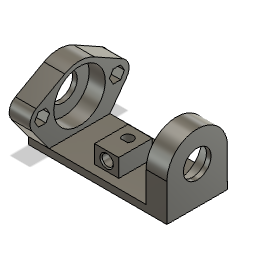
arm (Autodesk Fusion 360 design; units mm, degrees)
Autodesk Fusion 360 part; units mm, degrees
note: some values were not read from the file. Set by a fixed rule: which sketch regions a step uses.
sketch "Esquisse1" plane through (0, 0, 0) normal (0, 1, 0) x (1, 0, 0)
  circle A0 centre (0, 0) radius 2.25
  line L0 (30, -13.15) -> (-30, -13.15)
  line L1 (-30, -13.15) -> (-30, 13.15)
  line L2 (-30, 13.15) -> (30, 13.15)
  line L3 (30, 13.15) -> (30, -13.15)
  line L4 (30, -13.15) -> (-30, 13.15) construction
  line L5 (-30, -13.15) -> (30, 13.15) construction
  line L6 (-30, 13.15) -> (-21, 13.15)
  line L7 (-21, -13) -> (-30, -13)
  line L8 (-30, -13) -> (-30, 13.15)
  line L9 (0, 0) -> (0, -1.75) construction
  line L10 (0, -1.75) -> (1.4142, -1.75)
  line L11 (0, -1.75) -> (-1.4142, -1.75)
  dimension "d9" = 4.5
  dimension "d10" = 60
  dimension "d11" = 26.3
  dimension "d101" = 1.75
  constraint coincident A0.centre L9.start
  constraint horizontal L0
  constraint perpendicular L0 L1
  constraint parallel L0 L2
  constraint parallel L1 L3
  constraint coincident L4 A0.centre
  constraint coincident L5 A0.centre
  constraint horizontal L6
  constraint horizontal L7
  constraint vertical L8
  constraint vertical L9
  constraint coincident A0 L10.end
  constraint perpendicular L9 L10
  constraint symmetric L10.start L9 L11.start
  constraint symmetric L9 L10.end L11.end
  measures "d9" diameter of A0
  measures "d10" distance of L1.end L2.end
  measures "d11" distance of L0.end L1.end
  measures "d101" distance of A0.centre L9.end
ref_plane "Plan de construction1" through (30, 0, 0) normal (-1, 0, 0) x (0, 0, 1)
sketch "Esquisse2" plane through (30, 0, 0) normal (-1, 0, 0) x (0, 0, -1)
  line L0 (13, 0) -> (13, -20)
  line L1 (13.15, 0) -> (-13.15, 0)
  line L2 (-13.15, 0) -> (-13.15, -21)
  line L3 (0, 0) -> (0, -2) construction
  circle A0 centre (0, -13.15) radius 11.15
  circle A1 centre (0, -13.15) radius 6
  circle A2 centre (0, -13.15) radius 13.15
  dimension "d102" = 2
  dimension "d103" = 22.3
  dimension "d104" = 12
  dimension "d105" = 2
  constraint vertical L0
  constraint coincident L1.end L2.start
  constraint perpendicular L1 L2
  constraint coincident L3.start origin
  constraint perpendicular L1 L3
  constraint coincident L3.end A0
  constraint concentric A0 A1
  measures "d102" distance of L3.start L3.end
  measures "d103" diameter of A0
  measures "d104" diameter of A1
extrude "Extrusion1" add sketch "Esquisse2" along normal blind 9 contours L0 L1 A2 | L0 A2 | L1 L2 A2 picked at (12.3833, -13.15) makes body 1
extrude "Extrusion2" add sketch "Esquisse2" along normal blind 2 contours A0 bodies 1
ref_plane "Plan de construction2" through (-30, 0, 0) normal (1, 0, 0) x (0, 0, -1)
sketch "Esquisse16" plane through (-30, 0, 0) normal (1, 0, 0) x (0, 0, -1)
  circle A0 centre (0, 13.15) radius 13.15
  circle A1 centre (0, 13.15) radius 11.15
  circle A2 centre (0, 13.15) radius 6
  line L0 (13, 0) -> (13, 20)
  line L1 (-13.15, 0) -> (-13.15, 21)
  circle A3 centre (0, 13.15) radius 16.22 construction
  line L2 (0, 13.15) -> (-16.22, 13.15) construction
  line L3 (0, 13.15) -> (0, 29.37) construction
  circle A4 centre (-16.22, 13.15) radius 1.75
  circle A5 centre (-16.22, 13.15) radius 5.25
  circle A6 centre (16.22, 13.15) radius 5.25
  circle A7 centre (16.22, 13.15) radius 1.75
  line L4 (-13.15, 0) -> (-24.7417, 15.943)
  line L5 (0.9315, 28.726) -> (-24.187, 14.7182)
  line L6 (-0.9315, 28.726) -> (24.187, 14.7182)
  line L7 (13.15, 0) -> (24.7417, 15.943)
  line L8 (13.15, 0) -> (-13.15, 0)
  line L9 (-12.97, 13.1564) -> (-14.6006, 15.9678)
  line L10 (-14.6006, 15.9678) -> (-17.8506, 15.9614)
  line L11 (-17.8506, 15.9614) -> (-19.47, 13.1436)
  line L12 (-19.47, 13.1436) -> (-17.8394, 10.3322)
  line L13 (-17.8394, 10.3322) -> (-14.5894, 10.3386)
  line L14 (-14.5894, 10.3386) -> (-12.97, 13.1564)
  line L15 (14.6006, 15.9678) -> (17.8506, 15.9614)
  line L16 (12.97, 13.1564) -> (14.6006, 15.9678)
  line L17 (14.5894, 10.3386) -> (12.97, 13.1564)
  line L18 (17.8394, 10.3322) -> (14.5894, 10.3386)
  line L19 (19.47, 13.1436) -> (17.8394, 10.3322)
  line L20 (17.8506, 15.9614) -> (19.47, 13.1436)
  point P0 (-13, 0)
  point P1 (13.15, 0)
  point P2 (-16.22, 13.15)
  dimension "d106" = 32.44
  dimension "d107" = 3.5
  dimension "d108" = 3.5
  dimension "d124" = 3.25
  constraint concentric A1 A3
  constraint coincident A0.centre A1.centre
  constraint coincident A3 P2
  constraint perpendicular L1 L2
  constraint coincident A3 L3.end
  constraint perpendicular L2 L3
  constraint coincident P2 L2.end
  constraint symmetric L3 A4 A7
  constraint symmetric L3 A5 A6
  constraint coincident L1.start L4.start
  constraint tangent A5 L4
  constraint tangent A5 L5
  constraint tangent A0 L5
  constraint symmetric L3 L1.start P1
  constraint symmetric L3 L4.end L7.end
  constraint symmetric L3 L5.start L6.start
  constraint symmetric L3 L5.end L6.end
  constraint coincident P1 L7.start
  constraint symmetric L3 L9.start L16.start
  constraint symmetric L3 L9.end L15.start
  constraint symmetric L3 L10.end L15.end
  constraint symmetric L3 L11.end L19.start
  constraint symmetric L3 L12.end L18.start
  constraint symmetric L3 L13.end L17.start
  measures "d106" diameter of A3
  measures "d107" diameter of A4
  measures "d108" distance of A4
  measures "d124" distance of L9.start P2
extrude "Extrusion17" add sketch "Esquisse16" along normal blind 9 separate body contours A0 L0 L16 L17 | A0 L15 L16 L17 L18 L19 L20 | A0 L0 L16 | A0 L0 A6 L15 L16 L17 L18 L19 L20 | A0 L0 L17 | A0 A1 L0 A6 L16 L17 | A0 L0 A6 | L0 L16 L17 | A0 L0 A6 | A0 A1 A5 A6 | A0 A6 L6 | A0 L0 A6 L8 | A0 A1 A5 A6 | L0 A6 L7 L8 | A0 L1 A5 L8 | A0 L1 A5 L5 | A0 A1 A5 L9 L14 | A0 L1 A5 | L1 A5 L4 | A0 L1 A5 | L1 A5 L5 | A0 L1 L9 L10 L11 L12 L13 L14 | L1 A5 L9 L10 L11 L12 L13 L14 | A0 L1 L9 L14 makes body 2
extrude "Extrusion18" add sketch "Esquisse16" along normal blind 2 contours A1 A5 A6 | A1 A6 | A1 A5 bodies 2
extrude "Extrusion5" add sketch "Esquisse1" against normal blind 3 contours A0 L10 L11 | L0 L1 L2 L3 L6 L8 picked at (0.1016, -2.0764) bodies 1 2
sketch "Esquisse11" plane through (0, 0, 0) normal (0, 1, 0) x (-1, 0, 0)
  line L0 (-21, 13.15) -> (-21, -13)
  line L1 (-21, -13) -> (-30, -13)
  line L2 (21, 13.15) -> (-21, 13.15)
  line L3 (-2.25, 2.25) -> (2.25, 2.25)
  line L4 (2.25, 2.25) -> (2.25, -2.25)
  line L5 (2.25, -2.25) -> (-2.25, -2.25)
  line L6 (-2.25, -2.25) -> (-2.25, 2.25)
  line L7 (-2.25, 2.25) -> (2.25, -2.25) construction
  line L8 (2.25, 2.25) -> (-2.25, -2.25) construction
  line L9 (5.25, -5.25) -> (-5.25, -5.25)
  line L10 (-5.25, -5.25) -> (-5.25, 9.25)
  line L11 (-5.25, 9.25) -> (5.25, 9.25)
  line L12 (5.25, 9.25) -> (5.25, -5.25)
  arc A0 (-1.4142, 1.75) -> (1.4142, 1.75) centre (0, 0) ccw
  line L13 (-1.4142, 1.75) -> (1.4142, 1.75)
  line L14 (-30, -13) -> (-30, -13.15)
  line L15 (-30, -13.15) -> (21, -13.15)
  line L16 (21, -13.15) -> (21, 13.15)
  dimension "d65" = 4.5
  dimension "d66" = 4.5
  dimension "d92" = 3
  dimension "d93" = 7
  constraint horizontal L3
  constraint perpendicular L3 L4
  constraint parallel L3 L5
  constraint parallel L4 L6
  constraint coincident L7 A0.centre
  constraint coincident L8 A0.centre
  constraint coincident A0.centre origin
  constraint horizontal L9
  constraint vertical L10
  constraint horizontal L11
  constraint vertical L12
  measures "d65" distance of L4.end L5.end
  measures "d66" distance of L3.end L4.end
  measures "d92" distance of L5 L9
  measures "d93" distance of L3 L11
extrude "Extrusion13" add sketch "Esquisse11" along normal blind 7.8 contours L3 L4 L6 A0 L13 | L5 L6 A0 | L4 L5 A0 | L9 L10 L11 L12 bodies 1
sketch "Esquisse15" plane through (0, 0, 9.25) normal (0, 0, 1) x (1, 0, 0)
  line L0 (-5.25, 0) -> (5.25, 0)
  line L1 (5.25, 0) -> (5.25, 7.8)
  line L2 (5.25, 7.8) -> (-5.25, 7.8)
  line L3 (-5.25, 7.8) -> (-5.25, 0)
  line L4 (-5.25, 7.8) -> (5.25, 0) construction
  circle A0 centre (0, 3.9) radius 1.75
  circle A1 centre (0, 3.9) radius 2.4
  dimension "d96" = 3.5
  dimension "d120" = 4.8
  constraint coincident L2.end L3.start
  constraint coincident L0.end L1.start
  constraint midpoint L4 A0.centre
  constraint concentric A0 A1
  measures "d96" diameter of A0
  measures "d120" diameter of A1
extrude "Extrusion22" cut sketch "Esquisse15" against normal blind 5 contours A0 | A1 bodies 1
extrude "Extrusion16" cut sketch "Esquisse15" against normal blind 8 contours A0 bodies 1
chamfer "Chanfrein4" distance 0.5 angle 45 1 edges at (-2.2376, 4.7679, 9.25) on bodies 1
sketch "Esquisse18" plane through (-21, 0, 0) normal (1, 0, 0) x (0, 0, -1)
  circle A0 centre (-16.22, 13.15) radius 1.75
  circle A1 centre (16.22, 13.15) radius 1.75
  arc A2 (20.4663, 10.0627) -> (18.7771, 17.7352) centre (16.22, 13.15) ccw
  line L0 (18.7771, 17.7352) -> (6.4048, 24.6348)
  arc A3 (6.4048, 24.6348) -> (-6.4047, 24.6349) centre (0, 13.15) ccw
  line L1 (-6.4047, 24.6349) -> (-18.777, 17.7352)
  arc A4 (-18.777, 17.7352) -> (-20.4663, 10.0627) centre (-16.22, 13.15) ccw
  line L2 (-20.4663, 10.0627) -> (-13.15, 0)
  line L3 (-13.15, 0) -> (13.15, 0)
  line L4 (13.15, 0) -> (20.4663, 10.0627)
  line L5 (14.6006, 15.9678) -> (17.8506, 15.9614)
  line L6 (17.8506, 15.9614) -> (19.47, 13.1436)
  line L7 (19.47, 13.1436) -> (17.8394, 10.3322)
  line L8 (17.8394, 10.3322) -> (14.5894, 10.3386)
  line L9 (14.5894, 10.3386) -> (12.97, 13.1564)
  line L10 (12.97, 13.1564) -> (14.6006, 15.9678)
  line L11 (-14.6006, 15.9678) -> (-17.8506, 15.9614)
  line L12 (-12.97, 13.1564) -> (-14.6006, 15.9678)
  line L13 (-14.5894, 10.3386) -> (-12.97, 13.1564)
  circle A5 centre (0, 13.15) radius 16.22
  line L14 (-19.47, 13.1436) -> (-17.8394, 10.3322)
  line L15 (-17.8506, 15.9614) -> (-19.47, 13.1436)
  line L16 (-17.8394, 10.3322) -> (-14.5894, 10.3386)
  circle A6 centre (0, 13.15) radius 11.15
extrude "Extrusion23" cut sketch "Esquisse18" against normal blind 5 contours A0 L11 L12 L13 A5 L16 | A0 L11 A5 L14 L15 L16 | A1 L5 L8 L9 L10 A5 | A1 L5 L6 L7 L8 A5 bodies 1
split "Scinder11" [suppressed]
split "Scinder9" [suppressed]
split "Scinder10" [suppressed]
equation "bearing_outer_diam = 22.3 mm"
equation "bearing_depth = 7 mm"
equation "wall = 2 mm"
equation "bearing_inner_diam = 12 mm"
equation "m3_insert_hole = 5 mm"
equation "diam_screws = 32.44 mm"
equation "arm_len = 60 mm"
equation "motor_axle_diam = 4.5 mm"
equation "d9 = motor_axle_diam"
equation "d10 = arm_len"
equation "d11 = bearing_outer_diam + wall * 2"
equation "d16 = bearing_depth + wall"
equation "d18 = wall"
equation "d32 = -wall - 1 mm"
equation "shaft_above = 5 mm"
equation "insert_wall = 3 mm"
equation "shaft_insert_len = 5 mm"
equation "shaft_insert_od = 4.8 mm"
equation "m3_hole = 3.5 mm"
equation "shaft_insert_wall = 2 mm"
equation "d65 = motor_axle_diam"
equation "d66 = motor_axle_diam"
equation "shaft_coupling_wall = 2 mm"
equation "hex_nut_depth = 3 mm"
equation "hex_nut_diam = 6.5 mm"
equation "d75 = shaft_insert_od + shaft_insert_wall + 1 mm"
equation "bearing_offset = 2 mm"
equation "d92 = shaft_coupling_wall + 1 mm"
equation "d93 = shaft_coupling_wall + shaft_insert_len"
equation "d96 = m3_hole"
equation "d_shaft_diam = 3.5 mm"
equation "d101 = d_shaft_diam / 2"
equation "d102 = bearing_offset"
equation "d103 = bearing_outer_diam"
equation "d104 = bearing_inner_diam"
equation "d105 = wall"
equation "d106 = diam_screws"
equation "d107 = m3_hole"
equation "d108 = hex_nut_diam / 2 + wall - m3_hole / 2"
equation "d109 = bearing_depth + wall"
equation "d111 = wall"
equation "d120 = shaft_insert_od"
equation "d121 = -shaft_insert_len"
equation "d125 = -hex_nut_depth + -2 mm"
